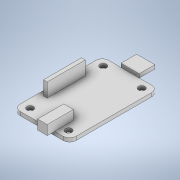
# Autodesk Inventor part: voice recognition
Saved by Autodesk Inventor 2020.2 (Build 242310000, 310)
## iProperties
Created: 2019-12-10
Part Number: voice recognition
Material: Generic
Document SubType Name: Modeling
Designer: athiy
Density: 1 g/cm^3
Appearance: Default
Author: athiy
Autodesk Inventor part; units mm, degrees
ref_plane "YZ Plane" through (0, 0, 0) normal (1, 0, 0) x (0, 1, 0)
ref_plane "XZ Plane" through (0, 0, 0) normal (0, 1, 0) x (-1, 0, 0)
ref_plane "XY Plane" through (0, 0, 0) normal (0, 0, 1) x (1, 0, 0)
sketch "Sketch1" plane through (0, 0, 0) normal (0, 1, 0) x (-1, 0, 0)
  line L0 (-3.5, 0) -> (-30, 0)
  line L1 (-30, -3.5) -> (-30, -44)
  line L2 (-26.5, -47.5) -> (-3.5, -47.5)
  line L3 (0, -44) -> (0, -3.5)
  line L4 (-26.5, 0) -> (-23.773, 0) construction
  circle A0 centre (-25.3298, -4.1188) radius 1.75
  circle A1 centre (-4.6702, -4.1188) radius 1.75
  circle A2 centre (-25.3298, -43.3812) radius 1.75
  circle A3 centre (-4.6702, -43.3812) radius 1.75
  arc A4 (0, -3.5) -> (-3.5, 0) centre (-3.5, -3.5) ccw
  arc A5 (-3.5, -47.5) -> (0, -44) centre (-3.5, -44) ccw
  arc A6 (-30, -44) -> (-26.5, -47.5) centre (-26.5, -44) ccw
  arc A7 (-26.5, 0) -> (-30, -3.5) centre (-26.5, -3.5) ccw
  point P0 (0, 0)
  point P1 (-30, -47.5)
  point P2 (0, -47.5)
  dimension "d0" = 30
  dimension "d1" = 47.5
  dimension "d4" = 3.5
  dimension "d5" = 3.5
  dimension "d6" = 3.5
  constraints: 10 end point, 8 centre point, 8 point on circle, 8 point on line, 8 tangent, 2 equal radius, 2 horizontal, 2 parallel, 1 perpendicular
  measures "d0" distance of point (0, -47.5) point (-30, -47.5)
  measures "d1" distance of point (-30, -47.5) L0.end
  measures "d4" diameter of A0
  measures "d5" radius of A4
  measures "d6" radius of A5
extrude "Extrusion1" add sketch "Sketch1" along normal blind 2
sketch "Sketch2" plane through (0, 2, 0) normal (0, 1, 0) x (1, 0, 0)
  line L0 (30, 0) -> (22, 0)
  line L1 (3.5, 0) -> (26.5, 0) projected
  line L2 (22, 0) -> (22, -4)
  line L3 (22, 0) -> (26, 0) construction
  line L4 (22, -4) -> (16.83, -4)
  line L5 (16.83, -4) -> (16.83, 10)
  line L6 (16.83, 10) -> (22, 10)
  line L7 (22, 10) -> (22, 0)
  point P0 (0, 0)
  dimension "d9" = 8
  dimension "d12" = 4
  dimension "d13" = 90
  dimension "d14" = 5.17
  dimension "d15" = 14
  constraints: 14 end point, 5 perpendicular, 1 horizontal, 1 point on line, 1 vertical
  measures "d9" distance of L0.start L0.end
  measures "d12" distance of L0.end L2.end
  measures "d13" angle of L2 L3
  measures "d14" distance of L2.end L4.end
  measures "d15" distance of L4.end L5.end
extrude "Extrusion2" add sketch "Sketch2" along normal blind 5.17
sketch "Sketch3" plane through (0, 2, 0) normal (0, 1, 0) x (1, 0, 0)
  line L0 (26.5, 47.5) -> (3.5, 47.5) projected
  line L1 (15, 47.5) -> (10.1, 47.5)
  line L2 (10.1, 47.5) -> (10.1, 55.9)
  line L3 (10.1, 55.9) -> (19.9, 55.9)
  line L4 (19.9, 55.9) -> (19.9, 47.5)
  point P0 (0, 0)
  dimension "d18" = 4.9
  dimension "d19" = 8.4
  dimension "d20" = 9.8
  constraints: 8 end point, 2 perpendicular, 2 point on line, 1 midpoint, 1 vertical
  measures "d18" distance of L1.start L1.end
  measures "d19" distance of L1.end L2.end
  measures "d20" distance of L2.end L3.end
extrude "Extrusion3" add sketch "Sketch3" along normal blind 2
sketch "Sketch4" plane through (0, 2, 0) normal (0, 1, 0) x (1, 0, 0)
  arc A0 (3.5, 47.5) -> (0, 44) centre (3.5, 44) ccw projected
  line L0 (0, 44) -> (0, 3.5) projected
  arc A1 (0, 3.5) -> (3.5, 0) centre (3.5, 3.5) ccw projected
  line L1 (3.5, 0) -> (3.5, 13.452)
  line L2 (3.5, 13.452) -> (2.5, 13.452)
  line L3 (10.1, 47.5) -> (3.5, 47.5) projected
  line L4 (3.5, 47.5) -> (3.5, 33.953)
  line L5 (3.5, 33.953) -> (2.5, 33.953)
  line L6 (2.5, 33.953) -> (2.5, 13.452)
  line L7 (3.5, 13.452) -> (4.5, 13.452)
  line L8 (3.5, 33.953) -> (4.5, 33.953)
  line L9 (4.5, 33.953) -> (4.5, 13.452)
  point P0 (0, 0)
  dimension "d26" = 13.452
  dimension "d27" = 1
  dimension "d28" = 13.547
  dimension "d29" = 1
  dimension "d30" = 1
  constraints: 16 end point, 4 perpendicular, 2 vertical, 1 horizontal
  measures "d26" distance of L1.start L1.end
  measures "d27" distance of L1.end L2.end
  measures "d28" distance of L3.end L4.end
  measures "d29" distance of L4.end L5.end
  measures "d30" distance of L1.end L7.end
extrude "Extrusion4" add sketch "Sketch4" along normal blind 7.514 contours L8 L9 L7 L2 L6 L5
body "Solid1"
